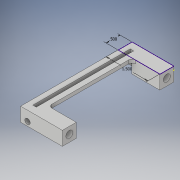
# Autodesk Inventor part: CarBrake
Saved by Autodesk Inventor 2018 (Build 220112000, 112)
## iProperties
Created: 2018-09-22
Part Number: CarBrake
Material: Generic
Document SubType Name: Modeling
Designer: Aditya Kendre
Density: 1 g/cm^3
Appearance: Default
Author: Aditya Kendre
Autodesk Inventor part; units mm, degrees
note: some values were not read from the file. Chosen so that the rebuilt part matches the saved one: edges of "Fillet1".
ref_plane "YZ Plane" through (0, 0, 0) normal (1, 0, 0) x (0, 1, 0)
ref_plane "XZ Plane" through (0, 0, 0) normal (0, 1, 0) x (-1, 0, 0)
ref_plane "XY Plane" through (0, 0, 0) normal (0, 0, 1) x (1, 0, 0)
sketch "Sketch1" plane through (0, 0, 0) normal (0, 1, 0) x (-1, 0, 0)
  line L0 (0, 0) -> (38.1, 0)
  line L1 (38.1, 0) -> (38.1, 12.7)
  line L2 (38.1, 12.7) -> (0, 12.7)
  line L3 (0, 12.7) -> (0, 0)
  dimension "d0" = 38.1
  dimension "d1" = 12.7
  constraints: 8 end point, 2 parallel, 1 horizontal, 1 perpendicular
  measures "d0" distance of L2.end L1.end
  measures "d1" distance of L1.end L0.end
sketch "Sketch2" plane through (0, 0, 0) normal (0, 0, 1) x (1, 0, 0)
  line L0 (0, 0) -> (-25.4, 0)
  line L1 (-25.4, 0) -> (-25.4, -12.7)
  line L2 (-25.4, -12.7) -> (0, -12.7)
  line L3 (0, -12.7) -> (0, 0)
  dimension "d2" = 25.4
  dimension "d3" = 12.7
  constraints: 8 end point, 2 parallel, 1 horizontal, 1 perpendicular
  measures "d2" distance of L2.end L1.end
  measures "d3" distance of L1.end L0.end
extrude "Extrusion1" add sketch "Sketch2" along normal blind 12.7
sketch "Sketch3" plane through (0, 0, 0) normal (0, 0, -1) x (-1, 0, 0)
  line L0 (0, 0) -> (25.4, 0) projected
  line L1 (25.4, 0) -> (38.1, 0)
  line L2 (38.1, 0) -> (38.1, -12.7)
  line L3 (38.1, -12.7) -> (25.4, -12.7)
  line L4 (25.4, -12.7) -> (25.4, 0)
  dimension "d6" = 12.7
  dimension "d7" = 12.7
  constraints: 8 end point, 2 parallel, 1 horizontal, 1 perpendicular
  measures "d6" distance of L2.end L3.end
  measures "d7" distance of L1.end L2.end
extrude "Extrusion2" add sketch "Sketch3" against normal blind 6.35
sketch "Sketch4" plane through (-25.4, 0, 12.7) normal (0, 1, 0) x (1, 0, 0)
  line L0 (-12.7, 12.7) -> (25.4, 12.7) projected
  line L1 (0, 12.7) -> (-12.7, 12.7)
  line L2 (-12.7, 12.7) -> (-12.7, -88.9)
  line L3 (-12.7, -88.9) -> (0, -88.9)
  line L4 (0, -88.9) -> (0, 12.7)
  dimension "d10" = 101.6
  constraints: 8 end point, 2 parallel, 1 horizontal, 1 perpendicular, 1 point on line
  measures "d10" distance of L2.end L1.end
extrude "Extrusion3" add sketch "Sketch4" against normal blind 3.175
sketch "Sketch5" plane through (-25.4, -3.175, 12.7) normal (0, -1, 0) x (1, 0, 0)
  point P0 (25.4, -12.7)
sketch "Sketch6" plane through (-38.1, 0, 101.6) normal (0, 0, 1) x (1, 0, 0)
  line L0 (12.7, -12.7) -> (38.1, -12.7) projected
  line L1 (0, 0) -> (38.1, 0)
  line L2 (38.1, 0) -> (38.1, -12.7)
  line L3 (38.1, -12.7) -> (0, -12.7)
  line L4 (0, -12.7) -> (0, 0)
  constraints: 8 end point, 2 parallel, 1 horizontal, 1 perpendicular
extrude "Extrusion4" add sketch "Sketch6" against normal blind 12.7
sketch "Sketch7" plane through (-38.1, 0, 88.9) normal (0, 0, -1) x (-1, 0, 0)
  line L0 (0, -12.7) -> (0, -3.175) projected
  line L1 (-12.7, -3.175) -> (0, -3.175) projected
  line L2 (0, -12.7) -> (-12.7, -12.7)
  line L3 (-12.7, -12.7) -> (-12.7, -3.175)
  line L4 (-12.7, -3.175) -> (0, -3.175)
  line L5 (0, -3.175) -> (0, -12.7)
  point P0 (-38.1, 0)
  constraints: 8 end point, 2 parallel, 1 horizontal, 1 perpendicular
extrude "Extrusion5" cut sketch "Sketch7" against normal blind 6.35
fillet "Fillet1" radius 3.175 2 edges at (-25.4, -1.5875, 12.7) (-25.4, -1.5875, 88.9)
sketch "Sketch8" plane through (-38.1, -12.7, 101.6) normal (0, 0, 1) x (1, 0, 0)
  point P0 (38.1, 12.7)
  point P1 (6.35, 3.81)
hole "Hole1" at (-31.75, -8.89, 101.6) direction (0, 0, -1) diameter 4.826 depth 107.95 tip angle 118
sketch "Sketch9" plane through (-25.4, -3.175, 12.7) normal (0, -1, 0) x (1, 0, 0)
  line L0 (-12.7, 82.55) -> (0, 82.55) projected
  line L1 (-4.7625, 82.55) -> (-7.9375, 82.55)
  line L2 (-7.9375, 82.55) -> (-7.9375, -6.35)
  line L3 (-7.9375, -6.35) -> (-4.7625, -6.35)
  line L4 (-4.7625, -6.35) -> (-4.7625, 82.55)
  point P0 (25.4, -12.7)
  point P1 (-6.35, 0)
  dimension "d25" = 3.175
  dimension "d26" = 88.9
  constraints: 8 end point, 2 parallel, 1 horizontal, 1 perpendicular, 1 point on line
  measures "d25" distance of L3.end L2.end
  measures "d26" distance of L2.end L1.end
extrude "Extrusion6" cut sketch "Sketch9" against normal blind 6.35
sketch "Sketch10" plane through (0, -12.7, 101.6) normal (1, 0, 0) x (0, 0, -1)
  line L0 (95.25, 9.525) -> (95.25, 0) projected
  point P0 (101.6, 12.7)
  point P1 (6.35, 6.35)
  point P2 (95.25, 6.35)
  constraints: 1 point on line
hole "Hole2" at (0, -6.35, 6.35) at (0, -6.35, 95.25) direction (-1, 0, 0) diameter 6.35 depth 12.7 tip angle 118
body "Solid1"
